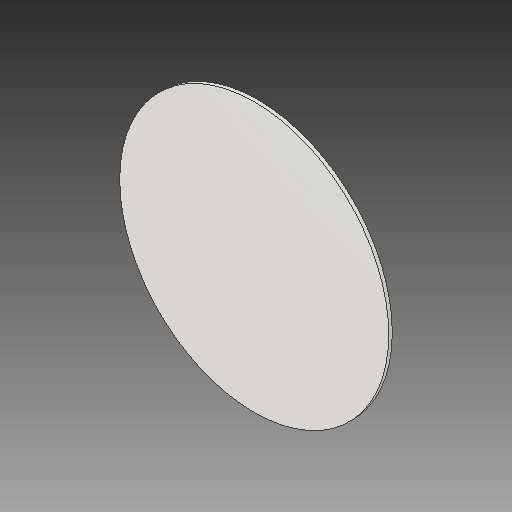
# Autodesk Inventor part: Burner
Saved by Autodesk Inventor 2019 (Build 230136000, 136)
## iProperties
Created: 2018-09-21
Part Number: Burner
Material: ABS Plastic
Document SubType Name: Modeling
Designer: user
Density: 1.06 g/cm^3
Appearance: Smooth - White
Author: user
Autodesk Inventor part; units mm, degrees
ref_plane "YZ Plane" through (0, 0, 0) normal (1, 0, 0) x (0, 1, 0)
ref_plane "XZ Plane" through (0, 0, 0) normal (0, 1, 0) x (-1, 0, 0)
ref_plane "XY Plane" through (0, 0, 0) normal (0, 0, 1) x (1, 0, 0)
sketch "Sketch1" plane through (0, 0, 0) normal (0, 0, 1) x (1, 0, 0)
  line L0 (-165.1, 165.1) -> (-165.1, -165.1) projected
  line L1 (-165.1, -165.1) -> (165.1, -165.1) projected
  line L2 (165.1, -165.1) -> (165.1, 165.1) projected
  line L3 (165.1, 165.1) -> (-165.1, 165.1) projected
  circle A0 centre (0, 0) radius 95.25
  dimension "d0" = 190.5
  constraints: 1 centre point, 1 coincident
  measures "d0" diameter of A0
extrude "Extrusion1" add sketch "Sketch1" along normal blind 2.54 contours A0
body "Solid1"
